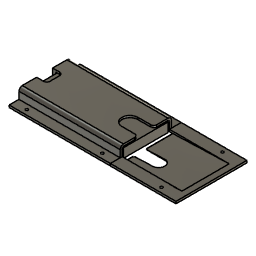
Battery Bank Bracket (Autodesk Fusion 360 design; units mm, degrees)
Autodesk Fusion 360 part; units mm, degrees
note: some values were not read from the file. Chosen so that the rebuilt part matches the saved one: which face or edge a step refers to.
sketch "Sketch1" plane through (0, 0, 0) normal (0, 0, 1) x (1, 0, 0)
  line L0 (24.0458, 15.1323) -> (173.1438, 15.1323)
  line L1 (173.1438, 15.1323) -> (173.1438, 83.2043)
  line L2 (173.1438, 83.2043) -> (24.0458, 83.2043)
  line L3 (24.0458, 83.2043) -> (24.0458, 15.1323)
  dimension "d1" = 149.098
  dimension "d2" = 68.072
  constraint horizontal L0
  constraint vertical L1
  constraint horizontal L2
  constraint vertical L3
  measures "d1" distance of L0.start L0.end
  measures "d2" distance of L0.start L2.end
extrude "Extrude1" add sketch "Sketch1" along normal blind 13.97 makes body 1
extrude "Extrude2" add 1 faces at (123.4445, 83.2043, 4.6567) along direction (0, 1, 0) blind 5 separate body on bodies 1 makes body 2
extrude "Extrude3" add 1 faces at (73.7451, 15.1323, 9.3133) along direction (0, -1, 0) blind 5 separate body on bodies 1 makes body 3
extrude "Extrude4" add 3 faces at (123.4445, 37.8229, 13.97) (73.7451, 13.4656, 13.97) (123.4445, 84.8709, 13.97) along direction (0, 0, 1) blind 5 separate body on bodies 1 2 3 makes body 4
combine "Combine1" operation add target body 2 tool bodies 3 4
extrude "Extrude5" add 2 faces at (24.0458, 60.5136, 4.6567) (24.0458, 60.5136, 17.3033) along direction (-1, 0, 0) blind 5 separate body on bodies 1 2 makes body 5
combine "Combine2" operation add target body 5 tool bodies 2
fillet "Fillet1" radius 5 2 edges at (96.0948, 88.2043, 18.97) (96.0948, 10.1323, 18.97) on bodies 5
move_face "OffsetFaces1" offset -2 3 faces at (73.7451, 15.1323, 9.3133) (123.4445, 83.2043, 4.6567) (123.4445, 37.8229, 13.97) on bodies 5
fillet "Fillet2" radius 2.5 2 edges at (98.5948, 13.1323, 15.97) (98.5948, 85.2043, 15.97) on bodies 5
sketch "Sketch2" plane through (0, 0, 18.97) normal (0, 0, 1) x (-1, 0, 0)
  line L0 (-19.0458, -15.1323) -> (-173.1438, -15.1323)
  line L1 (-173.1438, -15.1323) -> (-173.1438, -83.2043)
  line L2 (-173.1438, -83.2043) -> (-19.0458, -83.2043)
  line L3 (-19.0458, -83.2043) -> (-19.0458, -15.1323)
  circle A0 centre (-148.9617, -49.1683) radius 12.1464
  line L4 (-148.9617, -61.3147) -> (-173.1438, -61.3147)
  line L5 (-148.9617, -37.0219) -> (-173.1438, -37.0219)
  constraint coincident A0 L4.start
  constraint coincident L1 L4.end
  constraint tangent A0 L4
  constraint perpendicular L1 L4
  constraint coincident A0 L5.start
  constraint coincident L1 L5.end
  constraint tangent A0 L5
  constraint perpendicular L1 L5
extrude "Extrude6" cut sketch "Sketch2" against normal blind 3 contours L1 A0 L4 L5 | A0 bodies 5
fillet "Fillet3" radius 4.5 2 edges at (173.1438, 37.0219, 17.47) (173.1438, 61.3147, 17.47) on bodies 5
sketch "Sketch3" plane through (0, 88.2043, 0) normal (0, 1, 0) x (-1, 0, 0)
  line L0 (-19.0458, 13.97) -> (-173.1438, 13.97)
  line L1 (-173.1438, 13.97) -> (-173.1438, 0)
  line L2 (-173.1438, 0) -> (-19.0458, 0)
  line L3 (-19.0458, 0) -> (-19.0458, 13.97)
  line L4 (-173.1438, 3.2466) -> (-19.0458, 3.2466)
  constraint coincident L1 L4.start
  constraint coincident L3 L4.end
  constraint perpendicular L3 L4
extrude "Extrude7" add sketch "Sketch3" along normal blind 15 contours L1 L2 L3 L4 bodies 5
extrude "Extrude8" add 1 faces at (121.7778, 103.2043, 1.0822) along direction (0, -1, 0) blind 15 from surface at 93.072 on bodies 5 bodies 5
sketch "Sketch4" plane through (0, 0, 3.2466) normal (0, 0, 1) x (-1, 0, 0)
  line L0 (-19.0458, -88.2043) -> (-173.1438, -88.2043)
  line L1 (-173.1438, -88.2043) -> (-173.1438, -103.2043)
  line L2 (-173.1438, -103.2043) -> (-19.0458, -103.2043)
  line L3 (-19.0458, -103.2043) -> (-19.0458, -88.2043)
  point P0 (-38.526, -95.7043)
  point P1 (-153.526, -95.7043)
  point P2 (-38.526, -2.7043)
  point P3 (-153.526, -2.7043)
  dimension "d30" = -115
  dimension "d31" = 93
hole "Hole1" at (153.526, 2.7043, 3.2466) at (38.526, 2.7043, 3.2466) at (153.526, 95.7043, 3.2466) at (38.526, 95.7043, 3.2466) direction (0, 0, -1) diameter 4 depth 25 tip angle 118 bodies 5
sketch "Sketch5" plane through (0, 0, 18.97) normal (0, 0, 1) x (-1, 0, 0)
  arc A0 (-168.6438, -61.3147) -> (-173.1438, -65.8147) centre (-168.6438, -65.8147) ccw
  line L0 (-173.1438, -65.8147) -> (-173.1438, -83.2043)
  line L1 (-173.1438, -83.2043) -> (-19.0458, -83.2043)
  line L2 (-19.0458, -83.2043) -> (-19.0458, -15.1323)
  line L3 (-19.0458, -15.1323) -> (-173.1438, -15.1323)
  line L4 (-173.1438, -15.1323) -> (-173.1438, -32.5219)
  arc A1 (-173.1438, -32.5219) -> (-168.6438, -37.0219) centre (-168.6438, -32.5219) ccw
  line L5 (-168.6438, -37.0219) -> (-148.9617, -37.0219)
  arc A2 (-148.9617, -61.3147) -> (-148.9617, -37.0219) centre (-148.9617, -49.1683) ccw
  line L6 (-148.9617, -61.3147) -> (-168.6438, -61.3147)
  line L7 (-19.0458, -37.0219) -> (-50.0387, -37.0219)
  line L8 (-19.0458, -61.3147) -> (-50.0387, -61.3147)
  line L9 (-34.5423, -61.3147) -> (-34.5423, -37.0219)
  constraint coincident L2 L7.start
  constraint perpendicular L2 L7
  constraint coincident L2 L8.start
  constraint perpendicular L2 L8
  constraint midpoint L8 L9.start
  constraint midpoint L7 L9.end
  constraint perpendicular L7 L9
sketch "Sketch6" plane through (19.0458, 0, 0) normal (-1, 0, 0) x (0, -1, 0)
  arc A0 (-10.1323, 13.97) -> (-15.1323, 18.97) centre (-15.1323, 13.97) ccw
  line L0 (-15.1323, 18.97) -> (-83.2043, 18.97)
  arc A1 (-83.2043, 18.97) -> (-88.2043, 13.97) centre (-83.2043, 13.97) ccw
  line L1 (-88.2043, 13.97) -> (-88.2043, 3.2466)
  line L2 (-88.2043, 3.2466) -> (-103.2043, 3.2466)
  line L3 (-103.2043, 3.2466) -> (-103.2043, 0)
  line L4 (-103.2043, 0) -> (4.8677, 0)
  line L5 (4.8677, 0) -> (4.8677, 3.2466)
  line L6 (4.8677, 3.2466) -> (-10.1323, 3.2466)
  line L7 (-10.1323, 3.2466) -> (-10.1323, 13.97)
  line L8 (-61.3147, 18.97) -> (-37.0219, 18.97)
  line L9 (-37.0219, 18.97) -> (-37.0219, 11.102)
  line L10 (-37.0219, 11.102) -> (-61.3147, 11.102)
  line L11 (-61.3147, 11.102) -> (-61.3147, 18.97)
  point P0 (-61.3147, 18.97)
  constraint horizontal L8
  constraint vertical L9
  constraint horizontal L10
  constraint vertical L11
  constraint coincident P0 L8.start
extrude "Extrude9" cut sketch "Sketch5" against normal blind 14 contours L2 L7 L8 L9 bodies 5
fillet "Fillet4" radius 4.5 2 edges at (34.5423, 61.3147, 17.47) (34.5423, 37.0219, 17.47) on bodies 5
fillet "Fillet5" radius 2 2 edges at (21.5458, 61.3147, 4.97) (21.5458, 37.0219, 4.97) on bodies 5
sketch "Sketch7" plane through (173.1438, 0, 0) normal (1, 0, 0) x (0, 1, 0)
  line L0 (32.5219, 15.97) -> (32.5219, 18.97)
  line L1 (32.5219, 18.97) -> (15.1323, 18.97)
  arc A0 (15.1323, 18.97) -> (10.1323, 13.97) centre (15.1323, 13.97) ccw
  line L2 (10.1323, 13.97) -> (10.1323, 3.2466)
  line L3 (10.1323, 3.2466) -> (-4.8677, 3.2466)
  line L4 (-4.8677, 3.2466) -> (-4.8677, 0)
  line L5 (-4.8677, 0) -> (13.1323, 0)
  line L6 (13.1323, 0) -> (13.1323, 13.47)
  arc A1 (15.6323, 15.97) -> (13.1323, 13.47) centre (15.6323, 13.47) ccw
  line L7 (15.6323, 15.97) -> (32.5219, 15.97)
  line L8 (10.1323, 3.2466) -> (13.1323, 3.2466)
  constraint coincident L2.end L3.start
  constraint coincident L6 L8.end
  constraint perpendicular L6 L8
extrude "Extrude10" add sketch "Sketch7" along normal blind 100 contours L3 L4 L5 L6 L8 bodies 5
sketch "Sketch8" plane through (0, 13.1323, 0) normal (0, 1, 0) x (-1, 0, 0)
  line L0 (-24.0458, 13.47) -> (-173.1438, 13.47)
  line L1 (-173.1438, 13.47) -> (-173.1438, 3.2466)
  line L2 (-173.1438, 3.2466) -> (-273.1438, 3.2466)
  line L3 (-273.1438, 3.2466) -> (-273.1438, 0)
  line L4 (-273.1438, 0) -> (-24.0458, 0)
  line L5 (-24.0458, 0) -> (-24.0458, 13.47)
  line L6 (-173.1438, 3.2466) -> (-173.1438, 0)
  constraint coincident L1.end L2.start
  constraint coincident L4 L6.end
  constraint perpendicular L4 L6
extrude "Extrude11" add sketch "Sketch8" along normal blind 90.072 contours L2 L3 L4 L6 bodies 5
extrude "Extrude12" cut 1 faces at (173.1438, 37.1563, 2.1644) along direction (1, 0, 0) blind 5 on bodies 5 bodies 5
chamfer "Chamfer1" distance 86 distance2 3 1 edges at (178.1438, 49.1683, 3.2466) measured on face at (241.4771, 37.1563, 3.2466) on bodies 5
sketch "Sketch9" plane through (0.2079, 0, -5.9604) normal (-0.034863, 0, 0.999392) x (0, -1, 0)
  line L0 (-85.2043, 264.0964) -> (-85.2043, 178.0441)
  line L1 (-85.2043, 178.0441) -> (-13.1323, 178.0441)
  line L2 (-13.1323, 178.0441) -> (-13.1323, 264.0964)
  line L3 (-13.1323, 264.0964) -> (-85.2043, 264.0964)
  line L4 (-44.0897, 178.0441) -> (-25.6893, 178.0441)
  line L5 (-25.6893, 178.0441) -> (-25.6893, 221.561)
  line L6 (-25.6893, 221.561) -> (-44.0897, 221.561)
  line L7 (-44.0897, 221.561) -> (-44.0897, 178.0441)
  circle A0 centre (-34.8895, 207.2781) radius 9.2002
  constraint horizontal L4
  constraint vertical L5
  constraint horizontal L6
  constraint vertical L7
  constraint coincident L1 L4.start
  constraint tangent L5 A0
  constraint tangent L7 A0
extrude "Extrude13" cut sketch "Sketch9" against normal blind 15 contours L1 L4 L5 L7 A0 | A0 bodies 5
extrude "Extrude14" cut 1 faces at (178.1495, 37.9563, 0.0822) along direction (-0.999392, 0, -0.034863) blind 0.3 on bodies 5 bodies 5
fillet "Fillet6" radius 2 2 edges at (178.1438, 44.0897, 0.1233) (178.1438, 25.6893, 0.1233) on bodies 5
pattern_linear "R-Pattern1" count 2 spacing 90 along (1, 0, 0) count 2 spacing 93 along (0, 1, 0) of 1 faces at (153.0325, 4.6424, 2.1644) on bodies 5
sketch "Sketch10" plane through (0, 0, 3.2466) normal (0, 0, 1) x (-1, 0, 0)
  circle A0 centre (-243.526, -95.7043) radius 2
  circle A1 centre (-243.526, -2.7043) radius 2
  line L0 (-264.1438, -13.1323) -> (-173.1438, -13.1323)
  line L1 (-173.1438, -13.1323) -> (-173.1438, -10.1323)
  line L2 (-173.1438, -10.1323) -> (-19.0458, -10.1323)
  line L3 (-19.0458, -10.1323) -> (-19.0458, 4.8677)
  line L4 (-19.0458, 4.8677) -> (-273.1438, 4.8677)
  line L5 (-273.1438, 4.8677) -> (-273.1438, -103.2043)
  line L6 (-273.1438, -103.2043) -> (-19.0458, -103.2043)
  line L7 (-19.0458, -103.2043) -> (-19.0458, -88.2043)
  line L8 (-19.0458, -88.2043) -> (-173.1438, -88.2043)
  line L9 (-173.1438, -88.2043) -> (-173.1438, -85.2043)
  line L10 (-173.1438, -85.2043) -> (-264.1438, -85.2043)
  line L11 (-264.1438, -85.2043) -> (-264.1438, -13.1323)
  circle A2 centre (-38.526, -2.7043) radius 2
  circle A3 centre (-153.526, -2.7043) radius 2
  circle A4 centre (-153.526, -95.7043) radius 2
  circle A5 centre (-38.526, -95.7043) radius 2
  line L12 (-173.1438, -10.1323) -> (-173.1438, 4.8677)
  constraint coincident L1.end L2.start
  constraint coincident L4 L12.end
  constraint perpendicular L4 L12
split "Split1" by curves path "Sketch10" along L12 bodies 5 makes body 6 at (111.9604, 75.5068, 18.97)
